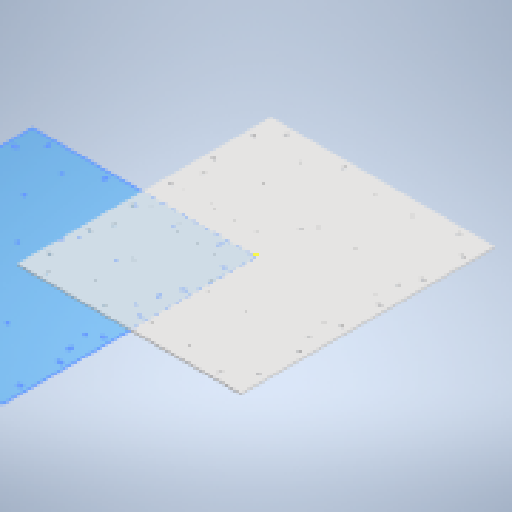
# Autodesk Inventor part: 발 받침대 받침_밑면
Saved by Autodesk Inventor 2024 (Build 280153000, 153)
## iProperties
Created: 2024-04-09
Part Number: 발 받침대 받침_밑면
Material: 일반
Document SubType Name: Modeling
Designer: ckhye
Density: 1 g/cm^3
Appearance: 기본값
Author: ckhye
Autodesk Inventor part; units mm, degrees
ref_plane "YZ Plane" through (0, 0, 0) normal (1, 0, 0) x (0, 1, 0)
ref_plane "XZ Plane" through (0, 0, 0) normal (0, 1, 0) x (-1, 0, 0)
ref_plane "XY Plane" through (0, 0, 0) normal (0, 0, 1) x (1, 0, 0)
sketch "스케치1" plane through (0, 0, 0) normal (0, 1, 0) x (-1, 0, 0)
  line L0 (195, 221) -> (-195, 221)
  line L1 (-195, 221) -> (-195, -221)
  line L2 (-195, -221) -> (195, -221)
  line L3 (195, -221) -> (195, 221)
  line L4 (195, 221) -> (-195, -221) construction
  line L5 (-195, 221) -> (195, -221) construction
  point P0 (0, 0)
  dimension "d0" = 390
  dimension "d1" = 442
  constraints: 12 end point, 2 midpoint, 2 parallel, 1 horizontal, 1 perpendicular
  measures "d0" distance of L2.end L1.end
  measures "d1" distance between parallel lines of L2 L0
extrude "돌출1" add sketch "스케치1" along normal blind 3
sketch "스케치4" plane through (0, 3, 0) normal (0, 1, 0) x (1, 0, 0)
  point P0 (0, 0)
sketch "스케치6" plane through (0, 3, 0) normal (0, 1, 0) x (1, 0, 0)
  line L0 (-303.9011, -178) -> (268.2048, -178)
  line L1 (-303.9011, 178) -> (283.641, 178)
  line L2 (-303.9011, 108) -> (283.641, 108)
  line L3 (-303.9011, -108) -> (268.2048, -108)
  line L4 (-155, -274.9581) -> (-155, 335.7384)
  line L5 (-55, -274.9581) -> (-55, 335.7384)
  line L6 (145, -274.9581) -> (145, 335.7384)
  line L7 (195, -221) -> (195, 221) projected
  line L8 (-195, 221) -> (-195, -221) projected
  line L9 (-195, -221) -> (195, -221) projected
  line L10 (195, 221) -> (-195, 221) projected
  line L11 (0, -22.8976) -> (0, 39.0777)
  line L12 (-29.975, 0) -> (33.4089, 0)
  line L13 (-184, 178) -> (-180, 178) construction
  line L14 (-184, 176) -> (-180, 176)
  line L15 (-180, 180) -> (-184, 180)
  arc A0 (-184, 180) -> (-184, 176) centre (-184, 178) ccw
  arc A1 (-180, 176) -> (-180, 180) centre (-180, 178) ccw
  line L16 (-184, 108) -> (-180, 108) construction
  line L17 (-184, 106) -> (-180, 106)
  line L18 (-180, 110) -> (-184, 110)
  arc A2 (-184, 110) -> (-184, 106) centre (-184, 108) ccw
  arc A3 (-180, 106) -> (-180, 110) centre (-180, 108) ccw
  line L19 (-184, -108) -> (-180, -108) construction
  line L20 (-184, -110) -> (-180, -110)
  line L21 (-180, -106) -> (-184, -106)
  arc A4 (-184, -106) -> (-184, -110) centre (-184, -108) ccw
  arc A5 (-180, -110) -> (-180, -106) centre (-180, -108) ccw
  line L22 (-184, -178) -> (-180, -178) construction
  line L23 (-184, -180) -> (-180, -180)
  line L24 (-180, -176) -> (-184, -176)
  arc A6 (-184, -176) -> (-184, -180) centre (-184, -178) ccw
  arc A7 (-180, -180) -> (-180, -176) centre (-180, -178) ccw
  line L25 (303.9011, -178) -> (-268.2048, -178)
  line L26 (303.9011, 178) -> (-283.641, 178)
  line L27 (303.9011, 108) -> (-283.641, 108)
  line L28 (303.9011, -108) -> (-268.2048, -108)
  line L29 (184, 178) -> (180, 178) construction
  line L30 (184, 176) -> (180, 176)
  line L31 (180, 180) -> (184, 180)
  arc A8 (184, 176) -> (184, 180) centre (184, 178) ccw
  arc A9 (180, 180) -> (180, 176) centre (180, 178) ccw
  line L32 (184, 108) -> (180, 108) construction
  line L33 (184, 106) -> (180, 106)
  line L34 (180, 110) -> (184, 110)
  arc A10 (184, 106) -> (184, 110) centre (184, 108) ccw
  arc A11 (180, 110) -> (180, 106) centre (180, 108) ccw
  line L35 (184, -108) -> (180, -108) construction
  line L36 (184, -110) -> (180, -110)
  line L37 (180, -106) -> (184, -106)
  arc A12 (184, -110) -> (184, -106) centre (184, -108) ccw
  arc A13 (180, -106) -> (180, -110) centre (180, -108) ccw
  line L38 (184, -178) -> (180, -178) construction
  line L39 (184, -180) -> (180, -180)
  line L40 (180, -176) -> (184, -176)
  arc A14 (184, -180) -> (184, -176) centre (184, -178) ccw
  arc A15 (180, -176) -> (180, -180) centre (180, -178) ccw
  line L41 (-155, -210) -> (-155, -206) construction
  line L42 (-153, -210) -> (-153, -206)
  line L43 (-157, -206) -> (-157, -210)
  arc A16 (-157, -210) -> (-153, -210) centre (-155, -210) ccw
  arc A17 (-153, -206) -> (-157, -206) centre (-155, -206) ccw
  line L44 (-55, -210) -> (-55, -206) construction
  line L45 (-53, -210) -> (-53, -206)
  line L46 (-57, -206) -> (-57, -210)
  arc A18 (-57, -210) -> (-53, -210) centre (-55, -210) ccw
  arc A19 (-53, -206) -> (-57, -206) centre (-55, -206) ccw
  line L47 (145, -210) -> (145, -206) construction
  line L48 (147, -210) -> (147, -206)
  line L49 (143, -206) -> (143, -210)
  arc A20 (143, -210) -> (147, -210) centre (145, -210) ccw
  arc A21 (147, -206) -> (143, -206) centre (145, -206) ccw
  line L50 (-155, 210) -> (-155, 206) construction
  line L51 (-153, 210) -> (-153, 206)
  line L52 (-157, 206) -> (-157, 210)
  arc A22 (-153, 210) -> (-157, 210) centre (-155, 210) ccw
  arc A23 (-157, 206) -> (-153, 206) centre (-155, 206) ccw
  line L53 (-55, 210) -> (-55, 206) construction
  line L54 (-53, 210) -> (-53, 206)
  line L55 (-57, 206) -> (-57, 210)
  arc A24 (-53, 210) -> (-57, 210) centre (-55, 210) ccw
  arc A25 (-57, 206) -> (-53, 206) centre (-55, 206) ccw
  line L56 (145, 210) -> (145, 206) construction
  line L57 (147, 210) -> (147, 206)
  line L58 (143, 206) -> (143, 210)
  arc A26 (147, 210) -> (143, 210) centre (145, 210) ccw
  arc A27 (143, 206) -> (147, 206) centre (145, 206) ccw
  line L59 (-273.1741, -32.5) -> (240.0899, -32.5)
  line L60 (-257.0626, 32.5) -> (240.0899, 32.5)
  line L61 (-184, -32.5) -> (-180, -32.5) construction
  line L62 (-184, -34.5) -> (-180, -34.5)
  line L63 (-180, -30.5) -> (-184, -30.5)
  arc A28 (-184, -30.5) -> (-184, -34.5) centre (-184, -32.5) ccw
  arc A29 (-180, -34.5) -> (-180, -30.5) centre (-180, -32.5) ccw
  line L64 (-184, 32.5) -> (-180, 32.5) construction
  line L65 (-184, 30.5) -> (-180, 30.5)
  line L66 (-180, 34.5) -> (-184, 34.5)
  arc A30 (-184, 34.5) -> (-184, 30.5) centre (-184, 32.5) ccw
  arc A31 (-180, 30.5) -> (-180, 34.5) centre (-180, 32.5) ccw
  line L67 (273.1741, -32.5) -> (-240.0899, -32.5)
  line L68 (257.0626, 32.5) -> (-240.0899, 32.5)
  line L69 (184, -32.5) -> (180, -32.5) construction
  line L70 (184, -34.5) -> (180, -34.5)
  line L71 (180, -30.5) -> (184, -30.5)
  arc A32 (184, -34.5) -> (184, -30.5) centre (184, -32.5) ccw
  arc A33 (180, -30.5) -> (180, -34.5) centre (180, -32.5) ccw
  line L72 (184, 32.5) -> (180, 32.5) construction
  line L73 (184, 30.5) -> (180, 30.5)
  line L74 (180, 34.5) -> (184, 34.5)
  arc A34 (184, 30.5) -> (184, 34.5) centre (184, 32.5) ccw
  arc A35 (180, 34.5) -> (180, 30.5) centre (180, 32.5) ccw
  line L75 (-289.5628, -68) -> (251.5599, -68)
  line L76 (-289.5628, 68) -> (251.5599, 68)
  line L77 (-170, -240.2082) -> (-170, 318.6302)
  line L78 (170, -254.5511) -> (170, 298.1594)
  line L79 (170, -80) -> (170, -76) construction
  line L80 (172, -80) -> (172, -76)
  line L81 (168, -76) -> (168, -80)
  arc A36 (168, -80) -> (172, -80) centre (170, -80) ccw
  arc A37 (172, -76) -> (168, -76) centre (170, -76) ccw
  line L82 (0, -80) -> (0, -76) construction
  line L83 (2, -80) -> (2, -76)
  line L84 (-2, -76) -> (-2, -80)
  arc A38 (-2, -80) -> (2, -80) centre (0, -80) ccw
  arc A39 (2, -76) -> (-2, -76) centre (0, -76) ccw
  line L85 (-170, -80) -> (-170, -76) construction
  line L86 (-168, -80) -> (-168, -76)
  line L87 (-172, -76) -> (-172, -80)
  arc A40 (-172, -80) -> (-168, -80) centre (-170, -80) ccw
  arc A41 (-168, -76) -> (-172, -76) centre (-170, -76) ccw
  line L88 (-170, 240.2082) -> (-170, -318.6302)
  line L89 (170, 254.5511) -> (170, -298.1594)
  line L90 (170, 80) -> (170, 76) construction
  line L91 (172, 80) -> (172, 76)
  line L92 (168, 76) -> (168, 80)
  arc A42 (172, 80) -> (168, 80) centre (170, 80) ccw
  arc A43 (168, 76) -> (172, 76) centre (170, 76) ccw
  line L93 (0, 80) -> (0, 76) construction
  line L94 (2, 80) -> (2, 76)
  line L95 (-2, 76) -> (-2, 80)
  arc A44 (2, 80) -> (-2, 80) centre (0, 80) ccw
  arc A45 (-2, 76) -> (2, 76) centre (0, 76) ccw
  line L96 (-170, 80) -> (-170, 76) construction
  line L97 (-168, 80) -> (-168, 76)
  line L98 (-172, 76) -> (-172, 80)
  arc A46 (-168, 80) -> (-172, 80) centre (-170, 80) ccw
  arc A47 (-172, 76) -> (-168, 76) centre (-170, 76) ccw
  circle A48 centre (-114.5, 39) radius 1.25
  circle A49 centre (-114.5, -19) radius 1.25
  circle A50 centre (-163.5, -19) radius 1.25
  circle A51 centre (-163.5, 39) radius 1.25
  circle A52 centre (-104, 32) radius 1.75
  circle A53 centre (-69, -32) radius 1.75
  circle A54 centre (-104, -32) radius 1.75
  circle A55 centre (-69, 32) radius 1.75
  circle A56 centre (-36, 36.5) radius 1.75
  circle A57 centre (-36, -36.5) radius 1.75
  circle A58 centre (162.5, -44) radius 1.75
  circle A59 centre (162.5, 44) radius 1.75
  point P0 (-182, 178)
  point P1 (-182, 108)
  point P2 (-182, -108)
  point P3 (-182, -178)
  point P4 (182, 178)
  point P5 (182, 108)
  point P6 (182, -108)
  point P7 (182, -178)
  point P8 (-155, -208)
  point P9 (-55, -208)
  point P10 (145, -208)
  point P11 (-155, 208)
  point P12 (-55, 208)
  point P13 (145, 208)
  point P14 (-182, -32.5)
  point P15 (-182, 32.5)
  point P16 (182, -32.5)
  point P17 (182, 32.5)
  point P18 (170, -78)
  point P19 (0, -78)
  point P20 (-170, -78)
  point P21 (170, 78)
  point P22 (0, 78)
  point P23 (-170, 78)
  dimension "d35" = 50
  dimension "d36" = 40
  dimension "d37" = 43
  dimension "d38" = 113
  dimension "d39" = 43
  dimension "d40" = 113
  dimension "d41" = 100
  dimension "d42" = 4
  dimension "d43" = 4
  dimension "d44" = 13
  dimension "d45" = 4
  dimension "d46" = 13
  dimension "d47" = 4
  dimension "d48" = 4
  dimension "d49" = 13
  dimension "d50" = 4
  dimension "d51" = 4
  dimension "d52" = 13
  dimension "d53" = 4
  dimension "d54" = 4
  dimension "d55" = 4
  dimension "d56" = 4
  dimension "d57" = 4
  dimension "d58" = 4
  dimension "d59" = 13
  dimension "d60" = 13
  dimension "d61" = 13
  dimension "d62" = 188.5
  dimension "d63" = 65
  dimension "d64" = 4
  dimension "d65" = 4
  dimension "d66" = 4
  dimension "d67" = 4
  dimension "d68" = 13
  dimension "d69" = 13
  dimension "d70" = 153
  dimension "d71" = 153
  dimension "d72" = 25
  dimension "d73" = 25
  dimension "d74" = 4
  dimension "d75" = 4
  dimension "d76" = 10
  dimension "d77" = 4
  dimension "d78" = 4
  dimension "d79" = 10
  dimension "d80" = 4
  dimension "d81" = 4
  dimension "d82" = 10
  dimension "d83" = 4
  dimension "d84" = 2.5
  dimension "d85" = 2.5
  dimension "d86" = 2.5
  dimension "d87" = 2.5
  dimension "d88" = 202
  dimension "d89" = 31.5
  dimension "d90" = 31.5
  dimension "d91" = 58
  dimension "d92" = 49
  dimension "d93" = 58
  dimension "d94" = 0
  dimension "d95" = 0
  dimension "d96" = 3.5
  dimension "d97" = 3.5
  dimension "d98" = 3.5
  constraints: 238 end point, 100 symmetric about line, 96 point on circle, 60 centre point, 48 tangent, 38 point on line, 13 parallel, 12 midpoint, 8 horizontal, 5 vertical, 2 perpendicular, 24 other
  measures "d35" distance between parallel lines of L7 L6
  measures "d36" distance between parallel lines of L8 L4
  measures "d37" distance between parallel lines of L9 L0
  measures "d38" distance between parallel lines of L9 L3
  measures "d39" distance between parallel lines of L10 L1
  measures "d40" distance between parallel lines of L10 L2
  measures "d41" distance between parallel lines of L4 L5
  measures "d42" distance of L13.start L13.end
  measures "d43" diameter of A1
  measures "d44" distance from line of L8 point (-182, 178)
  measures "d45" diameter of A3
  measures "d46" distance from line of L8 point (-182, 108)
  measures "d47" distance of L19.start L19.end
  measures "d48" diameter of A5
  measures "d49" distance from line of L8 point (-182, -108)
  measures "d50" distance of L22.start L22.end
  measures "d51" diameter of A7
  measures "d52" distance from line of L8 point (-182, -178)
  measures "d53" distance of L41.start L41.end
  measures "d54" diameter of A17
  measures "d55" distance of L44.start L44.end
  measures "d56" diameter of A19
  measures "d57" distance of L47.start L47.end
  measures "d58" diameter of A21
  measures "d59" distance from line of L9 point (145, -208)
  measures "d60" distance from line of L9 point (-55, -208)
  measures "d61" distance from line of L9 point (-155, -208)
  measures "d62" distance between parallel lines of L9 L59
  measures "d63" distance between parallel lines of L60 L59
  measures "d64" distance of L61.start L61.end
  measures "d65" diameter of A29
  measures "d66" distance of L64.start L64.end
  measures "d67" diameter of A31
  measures "d68" distance from line of L8 point (-182, 32.5)
  measures "d69" distance from line of L8 point (-182, -32.5)
  measures "d70" distance between parallel lines of L10 L76
  measures "d71" distance between parallel lines of L9 L75
  measures "d72" distance between parallel lines of L8 L77
  measures "d73" distance between parallel lines of L7 L78
  measures "d74" distance of L79.start L79.end
  measures "d75" diameter of A37
  measures "d76" distance from line of L75 point (170, -78)
  measures "d77" distance of L82.start L82.end
  measures "d78" diameter of A39
  measures "d79" distance from line of L75 point (0, -78)
  measures "d80" distance of L85.start L85.end
  measures "d81" diameter of A41
  measures "d82" distance from line of L75 point (-170, -78)
  measures "d83" distance of L16.start L16.end
  measures "d84" diameter of A48
  measures "d85" diameter of A49
  measures "d86" diameter of A50
  measures "d87" diameter of A51
  measures "d88" distance from line of L9 A50.centre
  measures "d89" distance from line of L8 A50.centre
  measures "d90" distance from line of L8 A51.centre
  measures "d91" distance of A50.centre A51.centre
  measures "d92" distance of A50.centre A49.centre
  measures "d93" vertical distance of A49.centre A51.centre
  measures "d94" vertical distance of A51.centre A48.centre
  measures "d95" horizontal distance of A49.centre A48.centre
  measures "d96" diameter of A52
  measures "d97" diameter of A53
  measures "d98" diameter of A54
extrude "돌출3" cut sketch "스케치6" against normal blind 10 contours A6 L24 A7 L0 | L0 A7 L23 A6 | A4 L21 A5 L3 | L3 A5 L20 A4 | A28 L63 A29 L59 | L59 A29 L62 A28 | A41 L86 A40 L77 | L77 A40 L87 A41 | A16 L43 A17 L4 | L4 A17 L42 A16 | A30 L66 A31 L60 | L60 A31 L65 A30 | A18 L46 A19 L5 | L5 A19 L45 A18 | A54 L59 | L59 A54 | A20 L49 A21 L6 | L6 A21 L48 A20 | A2 L18 A3 L2 | L2 A3 L17 A2 | A47 L98 A46 L77 | L77 A46 L97 A47 | A52 L60 | L60 A52 | A53 L59 | L59 A53 | A15 L40 A14 L0 | L0 A14 L39 A15 | A0 L15 A1 L1 | L1 A1 L14 A0 | A55 L60 | L60 A55 | A37 L80 A36 L78 | L78 A36 L81 A37 | A13 L37 A12 L3 | L3 A12 L36 A13 | A33 L71 A32 L59 | L59 A32 L70 A33 | A23 L52 A22 L4 | L4 A22 L51 A23 | A35 L74 A34 L60 | L60 A34 L73 A35 | A25 L55 A24 L5 | L5 A24 L54 A25 | A43 L92 A42 L78 | L78 A42 L91 A43 | A11 L34 A10 L2 | L2 A10 L33 A11 | A27 L58 A26 L6 | L6 A26 L57 A27 | A9 L31 A8 L1 | L1 A8 L30 A9 | A38 L84 A39 L83 | L94 A45 L95 A44 | A48 | A49 | A50 | A51 | A56 | A57 | A58 | A59
sketch "스케치7" plane through (0, 3, 0) normal (0, 1, 0) x (1, 0, 0)
  point P0 (0, 0)
sketch "스케치8" plane through (0, 3, 0) normal (0, 1, 0) x (1, 0, 0)
  circle A0 centre (77.5, -194) radius 2
  circle A1 centre (12.5, -194) radius 2
  circle A2 centre (12.5, -95) radius 2
  circle A3 centre (77.5, -95) radius 2
  line L0 (-195, -221) -> (195, -221) projected
  line L1 (195, -221) -> (195, 221) projected
  circle A4 centre (-101, -178) radius 2
  circle A5 centre (-101, -113) radius 2
  line L2 (-195, 221) -> (-195, -221) projected
  line L3 (25.1798, 0) -> (-29.0794, 0)
  circle A6 centre (77.5, 194) radius 2
  circle A7 centre (12.5, 194) radius 2
  circle A8 centre (12.5, 95) radius 2
  circle A9 centre (77.5, 95) radius 2
  circle A10 centre (-101, 178) radius 2
  circle A11 centre (-101, 113) radius 2
  point P0 (0, 0)
  dimension "d122" = 4
  dimension "d123" = 4
  dimension "d124" = 0
  dimension "d125" = 4
  dimension "d126" = 0
  dimension "d127" = 4
  dimension "d128" = 0
  dimension "d129" = 0
  dimension "d130" = 27
  dimension "d131" = 65
  dimension "d132" = 117.5
  dimension "d133" = 4
  dimension "d134" = 4
  dimension "d135" = 0
  dimension "d136" = 65
  dimension "d137" = 94
  dimension "d138" = 99
  dimension "d139" = 43
  constraints: 12 centre point, 6 symmetric about line, 2 end point, 1 horizontal, 6 other
  measures "d122" diameter of A0
  measures "d123" diameter of A1
  measures "d124" vertical distance of A0.centre A1.centre
  measures "d125" diameter of A2
  measures "d126" horizontal distance of A1.centre A2.centre
  measures "d127" diameter of A3
  measures "d128" vertical distance of A2.centre A3.centre
  measures "d129" horizontal distance of A0.centre A3.centre
  measures "d130" distance from line of L0 A0.centre
  measures "d131" distance of A1.centre A0.centre
  measures "d132" distance from line of L1 A0.centre
  measures "d133" diameter of A5
  measures "d134" diameter of A4
  measures "d135" horizontal distance of A5.centre A4.centre
  measures "d136" distance of A5.centre A4.centre
  measures "d137" distance from line of L2 A4.centre
  measures "d138" distance of A0.centre A3.centre
  measures "d139" distance from line of L0 A4.centre
extrude "돌출4" cut sketch "스케치8" against normal blind 10
